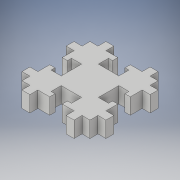
# Autodesk Inventor part: plunger_handle_center
Saved by Autodesk Inventor 2017 (Build 210142000, 142)
## iProperties
Created: 2017-01-19
Part Number: plunger_handle_center
Material: Generic
Document SubType Name: Modeling
Designer: John
Density: 1 g/cm^3
Appearance: Default
Author: John
Autodesk Inventor part; units mm, degrees
ref_plane "YZ Plane" through (0, 0, 0) normal (1, 0, 0) x (0, 1, 0)
ref_plane "XZ Plane" through (0, 0, 0) normal (0, 1, 0) x (-1, 0, 0)
ref_plane "XY Plane" through (0, 0, 0) normal (0, 0, 1) x (1, 0, 0)
sketch "Sketch2" plane through (0, 0, 0) normal (0, 1, 0) x (-1, 0, 0)
  line L0 (-7, 3.85) -> (-10.8, 3.85)
  line L1 (-12.8, 12.8) -> (-12.8, 9.8)
  line L2 (-10.8, 2.35) -> (-10.8, 3.85)
  line L3 (0, 0) -> (0, 7) construction
  line L4 (-12.8, 2.35) -> (-10.8, 2.35)
  line L5 (-7, 3.85) -> (-7, 0)
  line L6 (-7, 0) -> (0, 0) construction
  line L7 (-12.8, 9.8) -> (-15.8, 9.8)
  line L8 (-15.8, 9.8) -> (-15.8, 6.8)
  line L9 (-15.8, 6.8) -> (-12.8, 6.8)
  line L10 (-12.8, 6.8) -> (-12.8, 2.35)
  line L11 (-12.8, 12.8) -> (-9.8, 12.8)
  line L12 (-9.8, 12.8) -> (-9.8, 15.8)
  line L13 (-9.8, 15.8) -> (-6.8, 15.8)
  line L14 (-6.8, 15.8) -> (-6.8, 12.8)
  line L15 (0, 7) -> (-3.85, 7)
  line L16 (-3.85, 7) -> (-3.85, 10.8)
  line L17 (-3.85, 10.8) -> (-2.35, 10.8)
  line L18 (-2.35, 10.8) -> (-2.35, 12.8)
  line L19 (-2.35, 12.8) -> (-6.8, 12.8)
  line L20 (-7, -3.85) -> (-10.8, -3.85)
  line L21 (-12.8, -12.8) -> (-12.8, -9.8)
  line L22 (-10.8, -2.35) -> (-10.8, -3.85)
  line L23 (0, 0) -> (0, -7) construction
  line L24 (-12.8, -2.35) -> (-10.8, -2.35)
  line L25 (-7, -3.85) -> (-7, 0)
  line L26 (-12.8, -9.8) -> (-15.8, -9.8)
  line L27 (-15.8, -9.8) -> (-15.8, -6.8)
  line L28 (-15.8, -6.8) -> (-12.8, -6.8)
  line L29 (-12.8, -6.8) -> (-12.8, -2.35)
  line L30 (-12.8, -12.8) -> (-9.8, -12.8)
  line L31 (-9.8, -12.8) -> (-9.8, -15.8)
  line L32 (-9.8, -15.8) -> (-6.8, -15.8)
  line L33 (-6.8, -15.8) -> (-6.8, -12.8)
  line L34 (0, -7) -> (-3.85, -7)
  line L35 (-3.85, -7) -> (-3.85, -10.8)
  line L36 (-3.85, -10.8) -> (-2.35, -10.8)
  line L37 (-2.35, -10.8) -> (-2.35, -12.8)
  line L38 (-2.35, -12.8) -> (-6.8, -12.8)
  line L39 (7, 3.85) -> (10.8, 3.85)
  line L40 (12.8, 12.8) -> (12.8, 9.8)
  line L41 (10.8, 2.35) -> (10.8, 3.85)
  line L42 (12.8, 2.35) -> (10.8, 2.35)
  line L43 (7, 3.85) -> (7, 0)
  line L44 (7, 0) -> (0, 0) construction
  line L45 (12.8, 9.8) -> (15.8, 9.8)
  line L46 (15.8, 9.8) -> (15.8, 6.8)
  line L47 (15.8, 6.8) -> (12.8, 6.8)
  line L48 (12.8, 6.8) -> (12.8, 2.35)
  line L49 (12.8, 12.8) -> (9.8, 12.8)
  line L50 (9.8, 12.8) -> (9.8, 15.8)
  line L51 (9.8, 15.8) -> (6.8, 15.8)
  line L52 (6.8, 15.8) -> (6.8, 12.8)
  line L53 (0, 7) -> (3.85, 7)
  line L54 (3.85, 7) -> (3.85, 10.8)
  line L55 (3.85, 10.8) -> (2.35, 10.8)
  line L56 (2.35, 10.8) -> (2.35, 12.8)
  line L57 (2.35, 12.8) -> (6.8, 12.8)
  line L58 (7, -3.85) -> (10.8, -3.85)
  line L59 (3.85, -7) -> (3.85, -10.8)
  line L60 (2.35, -10.8) -> (2.35, -12.8)
  line L61 (3.85, -10.8) -> (2.35, -10.8)
  line L62 (7, -3.85) -> (7, 0)
  line L63 (0, -7) -> (3.85, -7)
  line L64 (2.35, -12.8) -> (6.8, -12.8)
  line L65 (9.8, -15.8) -> (6.8, -15.8)
  line L66 (6.8, -15.8) -> (6.8, -12.8)
  line L67 (9.8, -12.8) -> (9.8, -15.8)
  line L68 (12.8, -12.8) -> (9.8, -12.8)
  line L69 (12.8, -12.8) -> (12.8, -9.8)
  line L70 (10.8, -2.35) -> (10.8, -3.85)
  line L71 (12.8, -2.35) -> (10.8, -2.35)
  line L72 (12.8, -6.8) -> (12.8, -2.35)
  line L73 (12.8, -9.8) -> (15.8, -9.8)
  line L74 (15.8, -9.8) -> (15.8, -6.8)
  line L75 (15.8, -6.8) -> (12.8, -6.8)
  dimension "d4" = 2
  dimension "d8" = 3
  dimension "d9" = 3
  dimension "d11" = 3.8
  dimension "d13" = 3
  dimension "d14" = 3
  dimension "d15" = 3
  dimension "d16" = 3.85
  dimension "d17" = 3.85
  dimension "d18" = 3.8
  dimension "d20" = 2
  dimension "d22" = 3
  dimension "d23" = 3
  dimension "d27" = 2.35
  dimension "d28" = 2.35
  dimension "d29" = 7
  dimension "d30" = 7
  constraints: 156 end point, 53 symmetric about line, 6 parallel, 6 perpendicular, 5 horizontal, 4 coincident, 4 point on line, 3 vertical
  measures "d4" distance of L2.start L4.start
  measures "d8" distance of L9.end L1.end
  measures "d9" distance of L7.end L1.end
  measures "d11" distance of L0.end L0.start
  measures "d13" distance of L1.start L11.end
  measures "d14" distance of L11.end L12.end
  measures "d15" distance of L12.end L13.end
  measures "d16" distance of L0.start L5.end
  measures "d17" distance of L3.end L15.end
  measures "d18" distance of L15.end L16.end
  measures "d20" distance of L17.end L18.end
  measures "d22" distance of L13.end L14.end
  measures "d23" distance between parallel lines of L45 L49
  measures "d27" vertical distance of point (0, 0) L2.start
  measures "d28" horizontal distance of point (0, 0) L17.end
  measures "d29" distance between parallel lines of L3 L5
  measures "d30" distance between parallel lines of L6 L15
extrude "Extrusion1" add sketch "Sketch2" along normal mid plane 6
body "Solid1"
